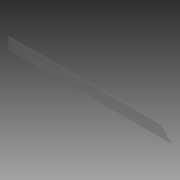
# Autodesk Inventor part: trapezoid polycarbonate ramp 125
Saved by Autodesk Inventor 2015 (Build 190159000, 159)
## iProperties
Created: 2015-01-20
Part Number: trapezoid polycarbonate ramp 125
Material: Polycarbonate, Clear
Document SubType Name: Modeling
Designer: Peter
Density: 1.2 g/cm^3
Appearance: Polycarbonate - Clear
Author: Peter
Autodesk Inventor part; units mm, degrees
ref_plane "YZ Plane" through (0, 0, 0) normal (1, 0, 0) x (0, 1, 0)
ref_plane "XZ Plane" through (0, 0, 0) normal (0, 1, 0) x (-1, 0, 0)
ref_plane "XY Plane" through (0, 0, 0) normal (0, 0, 1) x (1, 0, 0)
sketch "Sketch1" plane through (0, 0, 0) normal (0, 0, 1) x (1, 0, 0)
  line L0 (0, 0) -> (0, 137.16)
  line L1 (0, 137.16) -> (1828.8, 137.16)
  line L2 (1828.8, 137.16) -> (1965.96, 0)
  line L3 (1965.96, 0) -> (0, 0)
  dimension "d0" = 1828.8
  dimension "d1" = 137.16
  dimension "d2" = 137.16
  constraints: 8 end point, 1 parallel, 1 perpendicular, 1 vertical
  measures "d0" distance of L0.end L1.end
  measures "d1" horizontal distance of L2.end L1.end
  measures "d2" distance of L0.start L0.end
extrude "Extrusion1" add sketch "Sketch1" along normal blind 3.175
body "Solid1"
